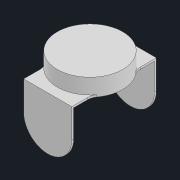
# Autodesk Inventor part: link4
Saved by Autodesk Inventor 2021 (Build 250183000, 183)
## iProperties
Created: 2021-07-10
Part Number: link4
Material: 一般
Document SubType Name: Modeling
Designer: yuta0
Density: 1 g/cm^3
Appearance: 既定
Author: yuta0
Autodesk Inventor part; units mm, degrees
ref_plane "YZ Plane" through (0, 0, 0) normal (1, 0, 0) x (0, 1, 0)
ref_plane "XZ Plane" through (0, 0, 0) normal (0, 1, 0) x (-1, 0, 0)
ref_plane "XY Plane" through (0, 0, 0) normal (0, 0, 1) x (1, 0, 0)
sketch "スケッチ1" plane through (0, 0, 0) normal (0, 1, 0) x (-1, 0, 0)
  line L0 (25, -44) -> (-25, -44)
  line L1 (-25, -44) -> (-25, 44)
  line L2 (-25, 44) -> (25, 44)
  line L3 (25, 44) -> (25, -44)
  line L4 (25, -44) -> (-25, 44) construction
  line L5 (-25, -44) -> (25, 44) construction
  point P0 (0, 0)
  dimension "d0" = 50
  dimension "d1" = 88
  constraints: 12 end point, 2 midpoint, 2 parallel, 1 horizontal, 1 perpendicular
  measures "d0" distance of L1.end L2.end
  measures "d1" distance of L0.end L1.end
extrude "押し出し1" add sketch "スケッチ1" against normal blind 2
sketch "スケッチ2" plane through (0, -2, 0) normal (0, -1, 0) x (1, 0, 0)
  line L0 (-25, 44) -> (-25, -44) projected
  line L1 (25, -44) -> (25, 44) projected
  line L2 (-25, -44) -> (25, -44)
  line L3 (25, -44) -> (25, -42)
  line L4 (25, -42) -> (-25, -42)
  line L5 (-25, -42) -> (-25, -44)
  line L6 (25, 44) -> (-25, 44) projected
  line L7 (-25, 44) -> (25, 44)
  line L8 (25, 44) -> (25, 42)
  line L9 (25, 42) -> (-25, 42)
  line L10 (-25, 42) -> (-25, 44)
  point P0 (0, 0)
  point P1 (-25, 42)
  point P2 (25, 42)
  point P3 (25, -44)
  dimension "d4" = 2
  dimension "d5" = 2
  constraints: 16 end point, 4 parallel, 2 horizontal, 2 perpendicular, 2 point on line
  measures "d4" distance between parallel lines of L6 L9
  measures "d5" distance between parallel lines of L2 L4
extrude "押し出し2" add sketch "スケッチ2" along normal blind 53 contours L6 L1 L9 L0 | L4 L1 L2 L0
sketch "スケッチ3" plane through (-25, 0, 44) normal (0, 0, 1) x (1, 0, 0)
  line L0 (0, 0) -> (50, 0) projected
  line L1 (0, 0) -> (0, -55) projected
  line L2 (50, -55) -> (0, -55) projected
  line L3 (50, 0) -> (50, -55) projected
  circle A0 centre (25, -30) radius 25
  line L4 (50, 0) -> (50, -55) projected
  point P0 (25, 0)
  point P1 (50, -30)
  point P2 (25, -55)
  point P3 (0, -30)
  constraints: 3 tangent, 1 centre point
extrude "押し出し3" cut sketch "スケッチ3" against normal through all contours A0 L2 L1 | L3 L2 A0
move or copy body "移動1" bodies to move or copy 1 copy no translate (0, 30, 0)
sketch "スケッチ4" plane through (-25, 28, 42) normal (0, -1, 0) x (1, 0, 0)
  circle A0 centre (25, -42) radius 34
  dimension "d14" = 68
  constraints: 1 centre point, 1 coincident
  measures "d14" diameter of A0
extrude "押し出し4" add sketch "スケッチ4" against normal blind 18
fillet "フィレット2" radius 12 4 edges at (25, 29, 23.0434) (25, 29, -23.0434) (-25, 29, 23.0434) (-25, 29, -23.0434)
